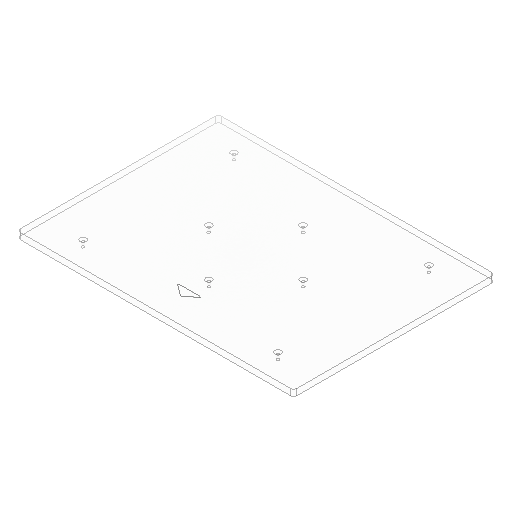
# Autodesk Inventor part: ICT-00-031
Saved by Autodesk Inventor 2026.1 (Build 301233020, 233B)
## iProperties
Company: Delta
Created: 2025-05-12
Part Number: ICT-00-031
Material: Acrílico TP
Document SubType Name: Modeling
Designer: Willian Pinheiro
Density: 1.19 g/cm^3
Appearance: Transparent - Clear
Description: Chapa T Fixação
Project: ICT
Mass: 1673 g
Surface Area: 2974.53 cm^2
Volume: 1405.88 cm^3
Acabamento: N/A
Dimensões: 10 x 320 x 440 mm
Total: 1
Author: Willian Pinheiro
Revision Number: 00
Title: ICT
Autodesk Inventor part; units mm, degrees
ref_plane "YZ Plane" through (0, 0, 0) normal (1, 0, 0) x (0, 1, 0)
ref_plane "XZ Plane" through (0, 0, 0) normal (0, 1, 0) x (-1, 0, 0)
ref_plane "XY Plane" through (0, 0, 0) normal (0, 0, 1) x (1, 0, 0)
sketch "Sketch1" plane through (0, 0, 0) normal (0, 0, 1) x (1, 0, 0)
  line L0 (-308, 0) -> (308, 0) construction
  line L1 (0, -224) -> (0, 224) construction
  line L2 (-220, 160) -> (220, 160)
  line L3 (220, 160) -> (220, -160)
  line L4 (220, -160) -> (-220, -160)
  line L5 (-220, -160) -> (-220, 160)
  line L6 (-20, -105) -> (0, -120)
  line L7 (-20, -105) -> (20, -105)
  line L8 (20, -105) -> (0, -120)
  point P0 (0, 0)
  point P1 (-155, 120)
  point P2 (-75, 0)
  point P3 (155, 120)
  point P4 (75, 0)
  point P5 (-155, -120)
  point P6 (155, -120)
  point P7 (-176, 110)
  point P8 (-146, 140)
  point P9 (176, 110)
  point P10 (146, 140)
  point P11 (-176, -110)
  point P12 (-146, -140)
  point P13 (146, -140)
  point P14 (176, -110)
  point P15 (-156, 0)
  point P16 (156, 0)
  point P17 (0, 75)
  point P18 (0, -75)
  dimension "d0" = 440
  dimension "d1" = 320
  dimension "d2" = 310
  dimension "d3" = 240
  dimension "d4" = 150
  dimension "d14" = 40
  dimension "d15" = 15
  dimension "d27" = 64
  dimension "d28" = 44
  dimension "d29" = 20
  dimension "d30" = 74
  dimension "d31" = 50
  dimension "d32" = 55
  dimension "d33" = 150
  constraints: 14 end point, 13 symmetric about line, 4 point on line, 2 parallel, 1 horizontal, 1 perpendicular, 2 other
  measures "d0" distance of L2.start L2.end
  measures "d1" distance of L4.end L2.start
  measures "d2" distance of point (155, 120) point (-155, 120)
  measures "d3" distance of point (-155, -120) point (-155, 120)
  measures "d4" distance of point (75, 0) point (-75, 0)
  measures "d14" distance of L6.start L7.end
  measures "d15" distance from line of L7 L6.end
  measures "d27" distance from line of point (-156, 0) L5
  measures "d28" distance from line of L5 point (-176, 110)
  measures "d29" distance from line of point (-146, 140) L2
  measures "d30" distance from line of point (-146, 140) L5
  measures "d31" distance from line of point (-176, 110) L2
  measures "d32" distance between parallel lines of L4 L7
  measures "d33" distance of point (0, -75) point (0, 75)
extrude "Extrusion1" add sketch "Sketch1" against normal blind 10 contours L2 L3 L4 L5 | L7 L8 L6
hole "Hole1" at (-75, 0, 0) at (75, 0, 0) at (155, 120, 0) at (155, -120, 0) at (-155, 120, 0) at (-155, -120, 0) at (0, -75, 0) at (0, 75, 0) direction (0, 0, -1) diameter 4.5 end through all countersink diameter 10 countersink angle 90 clearance for "Countersunk Flat Head Hex Socket Screw ISO 10642" size "M4" standard "ISO"
emboss "Emboss1" sketch "Sketch1" operation cut depth 0.1 direction (0, 0, -1) contours L7 L8 L6
fillet "Fillet1" radius 5 4 edges at (-220, -160, -5) (-220, 160, -5) (220, -160, -5) (220, 160, -5)
fillet "Fillet1" radius 1 3 edges at (-20, -105, -0.05) (0, -120, -0.05) (20, -105, -0.05)
body "Solid1"
